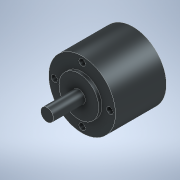
# Autodesk Inventor part: 775_gearhead
Saved by Autodesk Inventor 2022 (Build 260153000, 153)
## iProperties
Created: 2021-10-05
Part Number: 775_gearhead
Material: 鉄、ねずみ鋳鉄
Document SubType Name: Modeling
Designer: 中島 青蔵
Density: 7.15 g/cm^3
Appearance: 鉄 ねずみ鋳鉄
Author: 中島 青蔵
Autodesk Inventor part; units mm, degrees
ref_plane "YZ Plane" through (0, 0, 0) normal (1, 0, 0) x (0, 1, 0)
ref_plane "XZ Plane" through (0, 0, 0) normal (0, 1, 0) x (-1, 0, 0)
ref_plane "XY Plane" through (0, 0, 0) normal (0, 0, 1) x (1, 0, 0)
sketch "スケッチ1" plane through (0, 0, 0) normal (0, 0, 1) x (1, 0, 0)
  circle A0 centre (0, 0) radius 21
  dimension "d0" = 42
  constraints: 1 centre point, 1 coincident
  measures "d0" diameter of A0
extrude "押し出し1" add sketch "スケッチ1" along normal blind 32
sketch "スケッチ2" plane through (0, 0, 32) normal (0, 0, 1) x (1, 0, 0)
  circle A0 centre (0, 0) radius 12.5
  dimension "d3" = 25
  constraints: 1 centre point, 1 coincident
  measures "d3" diameter of A0
extrude "押し出し2" add sketch "スケッチ2" along normal blind 2
sketch "スケッチ3" plane through (0, 0, 34) normal (0, 0, 1) x (1, 0, 0)
  circle A0 centre (0, 0) radius 4
  dimension "d6" = 8
  constraints: 1 centre point, 1 coincident
  measures "d6" diameter of A0
extrude "押し出し3" add sketch "スケッチ3" along normal blind 20
sketch "スケッチ4" plane through (0, 0, 32) normal (0, 0, 1) x (1, 0, 0)
  point P0 (0, 0)
  point P1 (0, 17.5)
  point P2 (-17.5, 0)
  point P3 (0, -17.5)
  point P4 (17.5, 0)
  dimension "d9" = 17.5
  dimension "d12" = 360
  constraints: 5 other
  measures "d9" distance of point (0, 0) point (0, 17.5)
hole "穴1" at (0, 17.5, 32) at (-17.5, 0, 32) at (0, -17.5, 32) at (17.5, 0, 32) direction (0, 0, -1) diameter 4 depth 8 tip angle 118
